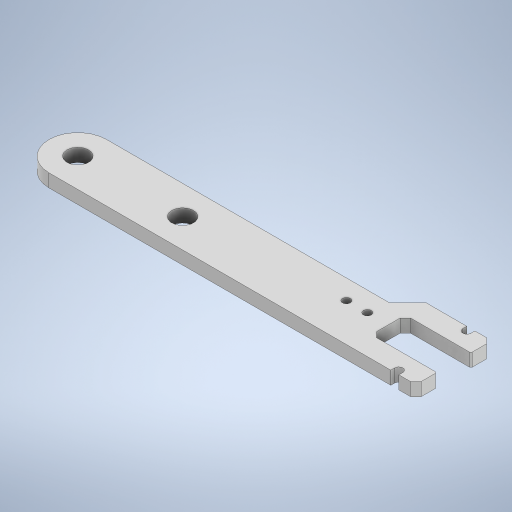
# Autodesk Inventor part: leg2
Saved by Autodesk Inventor 2024 (Build 280153000, 153)
## iProperties
Created: 2023-08-18
Part Number: leg2
Material: 常规
Document SubType Name: Modeling
Designer: wya
Density: 1 g/cm^3
Appearance: 默认
Author: wya
Autodesk Inventor part; units mm, degrees
ref_plane "YZ Plane" through (0, 0, 0) normal (1, 0, 0) x (0, 1, 0)
ref_plane "XZ Plane" through (0, 0, 0) normal (0, 1, 0) x (-1, 0, 0)
ref_plane "XY Plane" through (0, 0, 0) normal (0, 0, 1) x (1, 0, 0)
sketch "草图1" plane through (0, 0, 0) normal (0, 1, 0) x (-1, 0, 0)
  line L0 (0, 0) -> (140, 0)
  line L1 (140, 0) -> (140, -22)
  line L2 (140, -22) -> (0, -22)
  line L3 (0, -22) -> (0, 0)
  circle A0 centre (100, -11) radius 11
  circle A1 centre (100, -11) radius 4.15
  circle A2 centre (140, -11) radius 11
  circle A3 centre (140, -11) radius 4.15
  line L4 (25, -8) -> (0, -8)
  line L5 (0, -8) -> (0, -21)
  line L6 (0, -21) -> (25, -21)
  line L7 (25, -21) -> (25, -8)
  line L8 (32, -22) -> (0, -22)
  line L9 (0, -22) -> (0, -29)
  line L10 (0, -29) -> (32, -29)
  line L11 (32, -29) -> (32, -22)
  line L12 (32, -22) -> (25, -29)
  circle A4 centre (8, -1.55) radius 1.55
  line L13 (9.55, 0) -> (6.45, 0)
  line L14 (6.45, 0) -> (6.45, -1.55)
  line L15 (6.45, -1.55) -> (9.55, -1.55)
  line L16 (9.55, -1.55) -> (9.55, 0)
  circle A5 centre (33, -14.5) radius 1.525
  line L17 (25, -14.5) -> (20.7418, -14.5)
  circle A6 centre (41, -14.5) radius 1.525
  circle A7 centre (8, -27.45) radius 1.55
  line L18 (6.45, -27.45) -> (9.55, -27.45)
  line L19 (9.55, -27.45) -> (9.55, -29)
  line L20 (9.55, -29) -> (6.45, -29)
  line L21 (6.45, -29) -> (6.45, -27.45)
  point P0 (9.55, -1.55)
  point P1 (6.45, 0)
  point P2 (0, -8)
  point P3 (6.45, -29)
  dimension "d11" = 3.1
  dimension "d17" = 3.1
  dimension "d0" = 22
  dimension "d1" = 140
  dimension "d2" = 100
  dimension "d3" = 8.3
  dimension "d4" = 8.3
  dimension "d5" = 13
  dimension "d6" = 8
  dimension "d7" = 8
  dimension "d8" = 45
  dimension "d9" = 25
  dimension "d10" = 32
  dimension "d12" = 3.05
  dimension "d13" = 8
  dimension "d14" = 3.05
  dimension "d15" = 8
  dimension "d16" = 8
  constraints: 44 end point, 10 parallel, 8 horizontal, 7 point on line, 5 centre point, 5 perpendicular, 3 coincident, 3 midpoint, 3 vertical, 2 collinear, 2 tangent, 9 other
  measures "d0" distance between parallel lines of L2 L0
  measures "d1" distance between parallel lines of L3 L1
  measures "d2" distance from line of L3 A0.centre
  measures "d3" diameter of A1
  measures "d4" diameter of A3
  measures "d5" distance between parallel lines of L6 L4
  measures "d6" distance between parallel lines of L0 L4
  measures "d7" distance between parallel lines of L10 L6
  measures "d8" angle of L12 L11
  measures "d9" distance between parallel lines of L3 L7
  measures "d10" distance from line of L3 L8.start
  measures "d12" diameter of A5
  measures "d13" distance from line of L7 A5.centre
  measures "d14" diameter of A6
  measures "d15" distance of A5.centre A6.centre
  measures "d16" distance from line of L3 point (8, -1.55)
extrude "拉伸1" add sketch "草图1" along normal blind 5 contours L0 L14 A4 L16 A0 L2 L3 L6 L7 L4 | L2 L12 L10 L19 A7 L21 L9 | L0 A2 L2 A0 | A0 | A2 L1 A3 | L1 A3 A2
chamfer "倒角1" distance 2 angle 45 4 edges at (0, 2.5, 0) (-25, 2.5, -21) (0, 2.5, -29) (-25, 2.5, -8)
chamfer "倒角2" distance 0.5 angle 45 2 edges at (0, 2.5, -8) (0, 2.5, -21)
